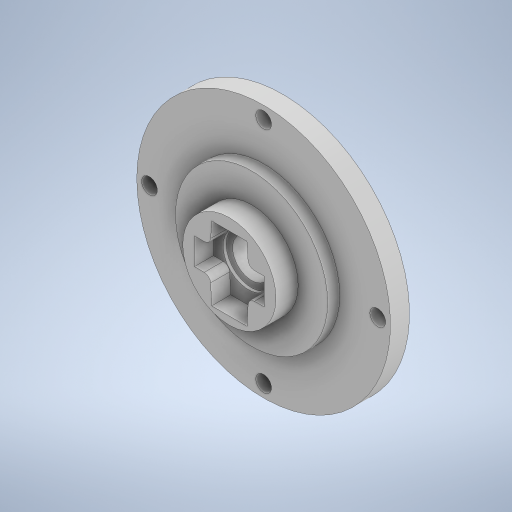
# Autodesk Inventor part: 180도 서보모터 십자축
Saved by Autodesk Inventor 2023.1 (Build 271208000, 208)
## iProperties
Created: 2021-08-22
Part Number: 180도 서보모터 십자축
Material: 일반
Document SubType Name: Modeling
Designer: fly01
Density: 1 g/cm^3
Appearance: 기본값
Author: fly01
Autodesk Inventor part; units mm, degrees
ref_plane "YZ Plane" through (0, 0, 0) normal (1, 0, 0) x (0, 1, 0)
ref_plane "XZ Plane" through (0, 0, 0) normal (0, 1, 0) x (-1, 0, 0)
ref_plane "XY Plane" through (0, 0, 0) normal (0, 0, 1) x (1, 0, 0)
sketch "스케치1" plane through (0, 0, 0) normal (0, 0, 1) x (1, 0, 0)
  circle A0 centre (0, 0) radius 2.5
  line L0 (-6.35, 0) -> (6.35, 0) construction
  line L1 (-6.35, -1.9) -> (6.35, -1.9)
  line L2 (6.35, 1.9) -> (-6.35, 1.9)
  arc A1 (-6.35, 1.9) -> (-6.35, -1.9) centre (-6.35, 0) ccw
  arc A2 (6.35, -1.9) -> (6.35, 1.9) centre (6.35, 0) ccw
  line L3 (0, 14.5) -> (0, -14.5) construction
  circle A3 centre (0, 14.5) radius 0.5
  circle A4 centre (0, -14.5) radius 0.5
  circle A5 centre (6.35, 0) radius 0.5
  circle A6 centre (-6.35, 0) radius 0.5
  circle A7 centre (-4.25, 0) radius 0.5
  circle A8 centre (4.25, 0) radius 0.5
  line L4 (0, -1.9) -> (0, -18.5)
  line L5 (0, 1.9) -> (0, 15.9)
  arc A9 (1.9954, 14.0355) -> (-1.9954, 14.0355) centre (0, 13.9) ccw
  arc A10 (-1.9969, -16.6117) -> (1.9969, -16.6117) centre (0, -16.5) ccw
  circle A11 centre (0, 0) radius 3.4
  line L6 (-1.9954, 14.0355) -> (-2.8196, 1.9)
  line L7 (1.9954, 14.0355) -> (2.8196, 1.9)
  line L8 (-2.8196, -1.9) -> (-1.9969, -16.6117)
  line L9 (2.8196, -1.9) -> (1.9969, -16.6117)
  circle A12 centre (0, 12.5) radius 0.5
  circle A13 centre (0, 10.5) radius 0.5
  circle A14 centre (0, 8.5) radius 0.5
  circle A15 centre (0, 6.5) radius 0.5
  circle A16 centre (0, 4.5) radius 0.5
  circle A17 centre (0, 0) radius 2.35
  circle A18 centre (0, -16.5) radius 0.5
  circle A19 centre (0, -12.5) radius 0.5
  circle A20 centre (0, -10.5) radius 0.5
  circle A21 centre (0, -8.5) radius 0.5
  circle A22 centre (0, -6.5) radius 0.5
  circle A23 centre (0, -4.5) radius 0.5
  dimension "d0" = 5
  dimension "d1" = 1.9
  dimension "d2" = 16.5
  dimension "d3" = 29
  dimension "d4" = 1
  dimension "d5" = 1
  dimension "d6" = 1
  dimension "d7" = 1
  dimension "d10" = 2.1
  dimension "d17" = 2.1
  dimension "d24" = 16.6
  dimension "d25" = 14
  dimension "d26" = 4
  dimension "d27" = 4
  dimension "d28" = 6.8
  dimension "d31" = 2
  dimension "d36" = 4.7
  dimension "d39" = 2
  dimension "d46" = 2
  constraints: 24 centre point, 22 end point, 14 point on circle, 10 point on line, 9 coincident, 8 tangent, 4 midpoint, 4 vertical, 3 horizontal, 1 parallel, 26 other
  measures "d0" diameter of A0
  measures "d1" radius of A2
  measures "d3" distance of L3.start L3.end
  measures "d4" diameter of A3
  measures "d5" diameter of A4
  measures "d6" diameter of A5
  measures "d7" diameter of A6
  measures "d10" distance of A6.centre A7.centre
  measures "d17" distance of A5.centre A8.centre
  measures "d24" distance of L4.start L4.end
  measures "d25" distance of L5.start L5.end
  measures "d26" diameter of A9
  measures "d27" diameter of A10
  measures "d28" diameter of A11
  measures "d31" distance of A3.centre A12.centre
  measures "d36" diameter of A17
  measures "d39" distance of A4.centre A18.centre
  measures "d46" distance of A4.centre A19.centre
extrude "돌출1" add sketch "스케치1" along normal blind 2.2 contours A0 L1 A17 L2 | A0 L2 A11 L1 | L2 A17 L5 A0 | A0 L5 A11 L2 | L1 A11 L4 A0 | A0 L4 A17 L1 | L5 A17 L2 A0 | A0 L2 A11 L5 | A17 L1 L2 | L2 L5 A17 | L4 A11 L1 A0 | A0 L1 A17 L4 | A17 L4 L1 | L2 A17 L1 A0 | A0 L1 A11 L2 | L5 L2 A17 | A17 L1 L4
extrude "돌출2" add sketch "스케치1" against normal blind 2.11 contours A0 L1 A17 L2 | A0 L2 A11 L1 | L2 A17 L5 A0 | A0 L5 A11 L2 | L1 A11 L4 A0 | A0 L4 A17 L1 | L5 A17 L2 A0 | A0 L2 A11 L5 | L2 A2 L1 A11 | A11 L5 A16 A15 A14 A13 A12 A3 A9 L7 | A17 L1 L2 | L2 L5 A17 | L4 A11 L1 A0 | A0 L1 A17 L4 | A17 L4 L1 | L9 A10 L4 A18 A4 A19 A20 A21 A22 A23 A11 | L2 A17 L1 A0 | A0 L1 A11 L2 | L5 L2 A17 | A11 L6 A9 L5 A3 A12 A13 A14 A15 A16 | A17 L1 L4 | L4 A23 A22 A21 A20 A19 A4 A18 A10 L8 A11 | A11 L1 A1 L2
extrude "돌출3" cut sketch "스케치1" along normal blind 3.65 contours A17 L1 L2 | L2 L5 A17 | A17 L4 L1 | L5 L2 A17 | A17 L1 L4
sketch "스케치2" plane through (0, 0, 0) normal (0, 0, 1) x (1, 0, 0)
  circle A0 centre (0, 0) radius 1.25
  dimension "d57" = 2.5
  constraints: 1 centre point, 1 coincident
  measures "d57" diameter of A0
extrude "돌출4" cut sketch "스케치2" against normal blind 7.6
sketch "스케치3" plane through (0, 0, -2.11) normal (0, 0, -1) x (-1, 0, 0)
  circle A0 centre (0, 0) radius 2.25
  dimension "d60" = 4.5
  constraints: 1 centre point, 1 coincident
  measures "d60" diameter of A0
extrude "돌출5" cut sketch "스케치3" against normal blind 1
sketch "스케치4" plane through (0, 0, -2.11) normal (0, 0, -1) x (-1, 0, 0)
  point P0 (0, 0)
sketch "스케치5" plane through (0, 0, -2.11) normal (0, 0, -1) x (-1, 0, 0)
  circle A0 centre (0, 0) radius 3.4
  circle A1 centre (0, 0) radius 2.25
  dimension "d63" = 4.5
  dimension "d64" = 6.8
  constraints: 2 centre point, 2 coincident
  measures "d63" diameter of A1
  measures "d64" diameter of A0
extrude "돌출6" add sketch "스케치5" along normal blind 0.4
sketch "스케치6" plane through (0, 0, -2.11) normal (0, 0, -1) x (-1, 0, 0)
  line L0 (0.9014, 15.3127) -> (-1.0592, 15.3127)
  line L1 (-1.0592, 15.3127) -> (-1.0592, 3.6394)
  line L2 (-1.0592, 3.6394) -> (0.9014, 3.6394)
  line L3 (0.9014, 3.6394) -> (0.9014, 15.3127)
  line L4 (1.0141, -3.7747) -> (-1.0592, -3.7747)
  line L5 (-1.0592, -3.7747) -> (-1.0592, -17.386)
  line L6 (-1.0592, -17.386) -> (1.0141, -17.386)
  line L7 (1.0141, -17.386) -> (1.0141, -3.7747)
  point P0 (0, 0)
  constraints: 16 end point, 4 parallel, 2 horizontal, 2 perpendicular, 1 point on line
extrude "돌출7" add sketch "스케치6" against normal blind 2.11
sketch "스케치7" plane through (0, 0, -2.11) normal (0, 0, -1) x (-1, 0, 0)
  circle A0 centre (0, 14.3) radius 0.5
  arc A1 (1.9954, 14.0355) -> (-1.9954, 14.0355) centre (0, 13.9) ccw projected
  line L0 (0, 0) -> (0, 0.7105)
  line L1 (0, 0) -> (0.8275, 0)
  circle A2 centre (0, 12.3) radius 0.5
  circle A3 centre (0, 10.3) radius 0.5
  circle A4 centre (0, 8.3) radius 0.5
  circle A5 centre (0, 6.3) radius 0.5
  circle A6 centre (0, 4.3) radius 0.5
  line L2 (0, 15.9) -> (3.4178, 15.9)
  arc A7 (1.9954, 14.0355) -> (-1.9954, 14.0355) centre (0, 13.9) ccw projected
  circle A8 centre (0, -16.9) radius 0.5
  arc A9 (-1.9969, -16.6117) -> (1.9969, -16.6117) centre (0, -16.5) ccw projected
  circle A10 centre (0, -14.9) radius 0.5
  circle A11 centre (0, -12.9) radius 0.5
  circle A12 centre (0, -10.9) radius 0.5
  circle A13 centre (0, -8.9) radius 0.5
  circle A14 centre (0, -6.9) radius 0.5
  circle A15 centre (0, -4.9) radius 0.5
  point P0 (0, -18.5)
  dimension "d69" = 1
  dimension "d73" = 2
  dimension "d78" = 1.6
  dimension "d79" = 1
  dimension "d80" = 1.6
  dimension "d86" = 2
  constraints: 13 centre point, 6 end point, 3 point on circle, 3 vertical, 2 horizontal, 1 tangent, 1 vertical alignment, 22 other
  measures "d69" diameter of A0
  measures "d73" distance of A0.centre A2.centre
  measures "d78" distance of A0.centre point (0, 15.9)
  measures "d79" diameter of A8
  measures "d80" distance of point (0, -18.5) A8.centre
  measures "d86" distance of A8.centre A10.centre
extrude "돌출8" cut sketch "스케치7" against normal blind 2.11
sketch "스케치9" plane through (0, 0, -2.11) normal (0, 0, -1) x (-1, 0, 0)
  circle A0 centre (0, 8.3) radius 0.5 projected
  line L0 (0.5, 8.3) -> (3.8465, 8.3)
  line L1 (3.8465, 8.3) -> (3.8465, 17.7965)
  line L2 (3.8465, 17.7965) -> (-4.3088, 17.7965)
  line L3 (-4.3088, 17.7965) -> (-4.3088, 8.3)
  line L4 (-4.3088, 8.3) -> (0.2806, 8.3)
  circle A1 centre (0, -8.9) radius 0.5 projected
  line L5 (0, -8.9) -> (5.2333, -8.9)
  line L6 (5.2333, -8.9) -> (5.2333, -19.7775)
  line L7 (5.2333, -19.7775) -> (-4.9031, -19.7775)
  line L8 (-4.9031, -19.7775) -> (-4.9031, -8.9)
  line L9 (-4.9031, -8.9) -> (0, -8.9)
  point P0 (0, 0)
  point P1 (0.5, -8.9)
  point P2 (-0.5, -8.9)
  point P3 (-0.5, 8.3)
  constraints: 20 end point, 7 perpendicular, 3 point on line, 2 horizontal, 2 other
extrude "돌출9" cut sketch "스케치9" against normal blind 10 contours A0 L4 L3 L2 L1 L0 | L5 L6 L7 L8 L9 A1
sketch "스케치10" plane through (0, 0, -2.11) normal (0, 0, -1) x (-1, 0, 0)
  line L0 (-0.0004, 7.8) -> (4.3151, 7.8)
  line L1 (4.3151, 7.8) -> (3.7805, 10.6296)
  line L2 (3.7805, 10.6296) -> (-3.3513, 10.6296)
  line L3 (-3.3513, 10.6296) -> (-3.4414, 7.8)
  line L4 (-3.4414, 7.8) -> (-0.0004, 7.8)
  arc A0 (-0.5, 8.3) -> (0.5, 8.3) centre (0, 8.3) ccw projected
  arc A1 (0.5, -8.9) -> (-0.5, -8.9) centre (0, -8.9) ccw projected
  line L5 (0, -8.4) -> (4.5069, -8.4)
  line L6 (4.5069, -8.4) -> (4.5069, -10.1694)
  line L7 (4.5069, -10.1694) -> (-4.0138, -10.1694)
  line L8 (-4.0138, -10.1694) -> (-4.0138, -8.4)
  line L9 (-4.0138, -8.4) -> (0, -8.4)
  point P0 (0, 0)
  constraints: 20 end point, 4 perpendicular, 2 horizontal, 2 point on line, 2 tangent, 1 collinear, 1 parallel, 1 point on circle
extrude "돌출10" cut sketch "스케치10" against normal blind 10
fillet "모깎기1" radius 2 4 edges at (2.4189, 7.8, -1.055) (-2.4189, 7.8, -1.055) (-2.4561, -8.4, -1.055) (2.4561, -8.4, -1.055)
sketch "스케치11" plane through (0, 0, -2.11) normal (0, 0, -1) x (-1, 0, 0)
  line L0 (-6.35, -1.9) -> (-2.8196, -1.9) projected
  line L1 (-2.8196, 1.9) -> (-6.35, 1.9) projected
  circle A0 centre (0, 6.3) radius 0.5 projected
  circle A1 centre (0, -6.9) radius 0.5 projected
  line L2 (2.8196, 1.9) -> (2.5455, 5.9355) projected
  line L3 (-2.5455, 5.9355) -> (-2.8196, 1.9) projected
  line L4 (0.5501, 7.8) -> (-0.5501, 7.8) projected
  line L5 (-2.8196, -1.9) -> (-2.5617, -6.5117) projected
  line L6 (2.5617, -6.5117) -> (2.8196, -1.9) projected
  point P0 (0, 0)
  point P1 (-4.5848, -1.9)
  point P2 (-4.5848, 1.9)
  point P3 (0, 7.8)
  dimension "d95" = 3.8
  dimension "d96" = 6.3
  dimension "d97" = 6.9
  dimension "d98" = 7.77
  dimension "d99" = 7.8
  dimension "d100" = 6.401
  constraints: 3 midpoint
  measures "d95" distance of point (-4.585, -1.9) point (-4.585, 1.9)
  measures "d96" distance of A0.centre point (0, 0)
  measures "d97" distance of A1.centre point (0, 0)
  measures "d98" angle of L2 L3
  measures "d99" distance of point (0, 0) point (0, 7.8)
  measures "d100" angle of L5 L6
sketch "스케치12" plane through (0, 0, -2.11) normal (0, 0, -1) x (-1, 0, 0)
  line L0 (2.5785, 5.3) -> (-2.5887, 5.3)
  line L1 (-2.5455, 5.9355) -> (-2.8196, 1.9) projected
  circle A0 centre (0, 4.3) radius 0.5 projected
  line L2 (3.3006, -5.9) -> (-2.5959, -5.9)
  line L3 (-2.8196, -1.9) -> (-2.5617, -6.5117) projected
  circle A1 centre (0, -4.9) radius 0.5 projected
  line L4 (2.8196, 1.9) -> (6.35, 1.9) projected
  line L5 (5.3, 1.9) -> (5.3, -1.9)
  circle A2 centre (4.25, 0) radius 0.5 projected
  line L6 (-6.35, 1.9) -> (-2.8196, 1.9) projected
  line L7 (-5.3, 1.9) -> (-5.3, -2.6397)
  circle A3 centre (-4.25, 0) radius 0.5 projected
  line L8 (5.3, 1.9) -> (9.4862, 1.9)
  line L9 (9.4862, 1.9) -> (9.4862, -2.8158)
  line L10 (9.4862, -2.8158) -> (5.3, -2.8158)
  line L11 (5.3, -2.8158) -> (5.3, 1.9)
  line L12 (3.3006, -5.9) -> (-3.636, -5.9)
  line L13 (-3.636, -5.9) -> (-3.636, -9.5734)
  line L14 (-3.636, -9.5734) -> (3.3006, -9.5734)
  line L15 (3.3006, -9.5734) -> (3.3006, -5.9)
  line L16 (-5.3, -2.6397) -> (-8.4677, -2.6397)
  line L17 (-8.4677, -2.6397) -> (-8.4677, 1.9)
  line L18 (-8.4677, 1.9) -> (-5.3, 1.9)
  line L19 (-5.3, 1.9) -> (-5.3, -2.6397)
  line L20 (-2.5887, 5.3) -> (3.3006, 5.3)
  line L21 (3.3006, 5.3) -> (3.3006, 8.0343)
  line L22 (3.3006, 8.0343) -> (-2.5887, 8.0343)
  line L23 (-2.5887, 8.0343) -> (-2.5887, 5.3)
  point P0 (0, 0)
  point P1 (-0.0051, 5.3)
  point P2 (-2.5617, -5.9)
  point P3 (-2.5959, -5.9)
  dimension "d101" = 1
  dimension "d102" = 1
  dimension "d104" = 1.05
  dimension "d105" = 1.05
  constraints: 40 end point, 8 parallel, 6 horizontal, 6 point on line, 4 perpendicular, 2 vertical, 1 midpoint
  measures "d101" distance of point (-0.005, 5.3) A0.centre
  measures "d102" distance from line of L2 A1.centre
  measures "d104" distance from line of L5 A2.centre
  measures "d105" distance from line of A3.centre L7
extrude "돌출11" cut sketch "스케치12" against normal blind 10 contours L0 L23 L22 L21 L20 | L15 L14 L13 L12 L2 | L4 L8 L9 L10 L11 L5 | L6 L7 L16 L17 L18
sketch "스케치14" plane through (0, 0, -2.11) normal (0, 0, -1) x (-1, 0, 0)
  line L0 (2.5887, 5.3) -> (-2.5887, 5.3) projected
  line L1 (-2.5887, 5.3) -> (-2.8196, 1.9) projected
  arc A0 (2.8196, 1.9) -> (-2.8196, 1.9) centre (0, 0) ccw projected
  line L2 (2.8196, 1.9) -> (2.5887, 5.3) projected
  circle A1 centre (0, 4.3) radius 0.5 projected
  circle A2 centre (0, 0) radius 3.4 projected
  circle A3 centre (0, 0) radius 2.25 projected
  line L3 (5.3, -1.9) -> (5.3, 1.9) projected
  line L4 (5.3, 1.9) -> (2.8196, 1.9) projected
  arc A4 (2.8196, -1.9) -> (2.8196, 1.9) centre (0, 0) ccw projected
  line L5 (2.8196, -1.9) -> (5.3, -1.9) projected
  circle A5 centre (4.25, 0) radius 0.5 projected
  line L6 (-2.5959, -5.9) -> (2.5959, -5.9) projected
  line L7 (2.5959, -5.9) -> (2.8196, -1.9) projected
  arc A6 (-2.8196, -1.9) -> (2.8196, -1.9) centre (0, 0) ccw projected
  line L8 (-2.8196, -1.9) -> (-2.5959, -5.9) projected
  circle A7 centre (0, -4.9) radius 0.5 projected
  line L9 (-5.3, 1.9) -> (-5.3, -1.9) projected
  line L10 (-5.3, -1.9) -> (-2.8196, -1.9) projected
  arc A8 (-2.8196, 1.9) -> (-2.8196, -1.9) centre (0, 0) ccw projected
  line L11 (-2.8196, 1.9) -> (-5.3, 1.9) projected
  circle A9 centre (-4.25, 0) radius 0.5 projected
  circle A10 centre (0, 0) radius 1.25 projected
  circle A11 centre (0, 0) radius 2.25 projected
  circle A12 centre (0, 0) radius 7.35
  point P0 (2.8196, -1.9)
  dimension "d111" = 14.7
  constraints: 1 centre point, 1 coincident
  measures "d111" diameter of A12
sketch "스케치15" plane through (0, 0, -2.51) normal (0, 0, -1) x (-1, 0, 0)
  line L0 (-8.2432, 8.5445) -> (15.2986, 8.5445)
  line L1 (15.2986, 8.5445) -> (15.2986, -14.1463)
  line L2 (15.2986, -14.1463) -> (-8.2432, -14.1463)
  line L3 (-8.2432, -14.1463) -> (-8.2432, 8.5445)
  point P0 (0, 0)
  constraints: 8 end point, 2 parallel, 1 horizontal, 1 perpendicular
extrude "돌출12" cut sketch "스케치15" along normal mid plane 10
extrude "돌출13" add sketch "스케치14" along normal blind 3 contours A12
sketch "스케치16" plane through (0, 0, -5.11) normal (0, 0, -1) x (-1, 0, 0)
  circle A0 centre (0, 0) radius 4
  circle A1 centre (0, 0) radius 7.35
  circle A2 centre (0, 0) radius 7.35 projected
  dimension "d114" = 8
  constraints: 2 centre point, 2 coincident, 1 concentric
  measures "d114" diameter of A0
extrude "돌출14" add sketch "스케치16" along normal blind 0.5
sketch "스케치17" plane through (0, 0, -2.11) normal (0, 0, 1) x (1, 0, 0)
  circle A0 centre (0, 0) radius 7.35 projected
  line L0 (2.5887, 5.3) -> (-2.5887, 5.3) projected
  line L1 (2.8196, 1.9) -> (2.5887, 5.3) projected
  line L2 (5.3, 1.9) -> (2.8196, 1.9) projected
  line L3 (5.3, -1.9) -> (5.3, 1.9) projected
  line L4 (2.8196, -1.9) -> (5.3, -1.9) projected
  line L5 (2.5959, -5.9) -> (2.8196, -1.9) projected
  line L6 (-2.5959, -5.9) -> (2.5959, -5.9) projected
  line L7 (-2.8196, -1.9) -> (-2.5959, -5.9) projected
  line L8 (-5.3, -1.9) -> (-2.8196, -1.9) projected
  line L9 (-5.3, 1.9) -> (-5.3, -1.9) projected
  line L10 (-2.8196, 1.9) -> (-5.3, 1.9) projected
  line L11 (-2.5887, 5.3) -> (-2.8196, 1.9) projected
  line L12 (-2.7755, 5.5) -> (2.7755, 5.5)
  line L13 (2.7755, 5.5) -> (3.0065, 2.1)
  line L14 (3.0065, 2.1) -> (5.5, 2.1)
  line L15 (5.5, 2.1) -> (5.5, -2.1)
  line L16 (5.5, -2.1) -> (3.0087, -2.1)
  line L17 (3.0087, -2.1) -> (2.785, -6.1)
  line L18 (2.785, -6.1) -> (-2.785, -6.1)
  line L19 (-2.785, -6.1) -> (-3.0087, -2.1)
  line L20 (-3.0087, -2.1) -> (-5.5, -2.1)
  line L21 (-5.5, -2.1) -> (-5.5, 2.1)
  line L22 (-5.5, 2.1) -> (-3.0065, 2.1)
  line L23 (-3.0065, 2.1) -> (-2.7755, 5.5)
  dimension "d117" = 0.2
  constraints: 24 end point, 11 other
  measures "d117" distance between parallel lines of L0 L12
extrude "돌출15" cut sketch "스케치17" against normal blind 3 contours L1 L2 L3 L4 L5 L6 L7 L8 L9 L10 L11 L0 | L12 L13 L14 L15 L16 L17 L18 L19 L20 L21 L22 L23
fillet "모깎기2" radius 1 4 edges at (-3.0065, 2.1, -3.61) (3.0065, 2.1, -3.61) (3.0087, -2.1, -3.61) (-3.0087, -2.1, -3.61)
sketch "스케치18" plane through (0, 0, -5.61) normal (0, 0, -1) x (-1, 0, 0)
  circle A0 centre (0, 0) radius 12
  dimension "d121" = 24
  constraints: 1 centre point, 1 coincident
  measures "d121" diameter of A0
extrude "돌출16" add sketch "스케치18" along normal blind 1.9
sketch "스케치19" plane through (0, 0, -7.51) normal (0, 0, -1) x (-1, 0, 0)
  circle A0 centre (0, 0) radius 20
  circle A1 centre (0, 18) radius 1.25
  circle A2 centre (-18, 0) radius 1.25
  circle A3 centre (0, -18) radius 1.25
  circle A4 centre (18, 0) radius 1.25
  dimension "d124" = 40
  dimension "d125" = 2.5
  dimension "d126" = 18
  dimension "d129" = 360
  constraints: 5 centre point, 1 coincident, 9 other
  measures "d124" diameter of A0
  measures "d125" diameter of A1
  measures "d126" distance of point (0, 0) A1.centre
extrude "돌출17" add sketch "스케치19" along normal blind 3
sketch "스케치20" plane through (0, 0, -5.61) normal (0, 0, 1) x (1, 0, 0)
  circle A0 centre (0, 0) radius 4 projected
  circle A1 centre (0, 0) radius 3
  dimension "d133" = 6
  constraints: 1 centre point, 1 coincident
  measures "d133" diameter of A1
extrude "돌출18" cut sketch "스케치20" against normal blind 16 contours A1
